Autodesk Fusion 360 part; units mm, degrees
note: some values were not read from the file. Chosen so that the rebuilt part matches the saved one: which pieces of a blend or face edit are solid.
(part 3 of 5)
  circle A747 centre (14.4118, -83.5294) radius 1.5
  circle A748 centre (21.3235, -83.5294) radius 1.5
  circle A749 centre (28.2353, -83.5294) radius 1.5
  circle A750 centre (35.1471, -83.5294) radius 1.5
  circle A751 centre (42.0588, -83.5294) radius 1.5
  circle A752 centre (48.9706, -83.5294) radius 1.5
  circle A753 centre (55.8824, -83.5294) radius 1.5
  circle A754 centre (62.7941, -83.5294) radius 1.5
  circle A755 centre (69.7059, -83.5294) radius 1.5
  circle A756 centre (76.6176, -83.5294) radius 1.5
  circle A757 centre (83.5294, -83.5294) radius 1.5
  circle A758 centre (90.4412, -83.5294) radius 1.5
  circle A759 centre (97.3529, -83.5294) radius 1.5
  circle A760 centre (104.2647, -83.5294) radius 1.5
  circle A761 centre (111.1765, -83.5294) radius 1.5
  circle A762 centre (118.0882, -83.5294) radius 1.5
  circle A763 centre (125, -83.5294) radius 1.5
  circle A764 centre (131.9118, -83.5294) radius 1.5
  circle A765 centre (138.8235, -83.5294) radius 1.5
  circle A766 centre (145.7353, -83.5294) radius 1.5
  circle A767 centre (152.6471, -83.5294) radius 1.5
  circle A768 centre (159.5588, -83.5294) radius 1.5
  circle A769 centre (166.4706, -83.5294) radius 1.5
  circle A770 centre (173.3824, -83.5294) radius 1.5
  circle A771 centre (180.2941, -83.5294) radius 1.5
  circle A772 centre (187.2059, -83.5294) radius 1.5
  circle A773 centre (194.1176, -83.5294) radius 1.5
  circle A774 centre (201.0294, -83.5294) radius 1.5
  circle A775 centre (207.9412, -83.5294) radius 1.5
  circle A776 centre (214.8529, -83.5294) radius 1.5
  circle A777 centre (221.7647, -83.5294) radius 1.5
  circle A778 centre (228.6765, -83.5294) radius 1.5
  circle A779 centre (235.5882, -83.5294) radius 1.5
  circle A780 centre (242.5, -83.5294) radius 1.5
  circle A781 centre (14.4118, -90.4412) radius 1.5
  circle A782 centre (21.3235, -90.4412) radius 1.5
  circle A783 centre (28.2353, -90.4412) radius 1.5
  circle A784 centre (35.1471, -90.4412) radius 1.5
  circle A785 centre (42.0588, -90.4412) radius 1.5
  circle A786 centre (48.9706, -90.4412) radius 1.5
  circle A787 centre (55.8824, -90.4412) radius 1.5
  circle A788 centre (62.7941, -90.4412) radius 1.5
  circle A789 centre (69.7059, -90.4412) radius 1.5
  circle A790 centre (76.6176, -90.4412) radius 1.5
  circle A791 centre (83.5294, -90.4412) radius 1.5
  circle A792 centre (90.4412, -90.4412) radius 1.5
  circle A793 centre (97.3529, -90.4412) radius 1.5
  circle A794 centre (104.2647, -90.4412) radius 1.5
  circle A795 centre (111.1765, -90.4412) radius 1.5
  circle A796 centre (118.0882, -90.4412) radius 1.5
  circle A797 centre (125, -90.4412) radius 1.5
  circle A798 centre (131.9118, -90.4412) radius 1.5
  circle A799 centre (138.8235, -90.4412) radius 1.5
  circle A800 centre (145.7353, -90.4412) radius 1.5
  circle A801 centre (152.6471, -90.4412) radius 1.5
  circle A802 centre (159.5588, -90.4412) radius 1.5
  circle A803 centre (166.4706, -90.4412) radius 1.5
  circle A804 centre (173.3824, -90.4412) radius 1.5
  circle A805 centre (180.2941, -90.4412) radius 1.5
  circle A806 centre (187.2059, -90.4412) radius 1.5
  circle A807 centre (194.1176, -90.4412) radius 1.5
  circle A808 centre (201.0294, -90.4412) radius 1.5
  circle A809 centre (207.9412, -90.4412) radius 1.5
  circle A810 centre (214.8529, -90.4412) radius 1.5
  circle A811 centre (221.7647, -90.4412) radius 1.5
  circle A812 centre (228.6765, -90.4412) radius 1.5
  circle A813 centre (235.5882, -90.4412) radius 1.5
  circle A814 centre (242.5, -90.4412) radius 1.5
  circle A815 centre (14.4118, -97.3529) radius 1.5
  circle A816 centre (21.3235, -97.3529) radius 1.5
  circle A817 centre (28.2353, -97.3529) radius 1.5
  circle A818 centre (35.1471, -97.3529) radius 1.5
  circle A819 centre (42.0588, -97.3529) radius 1.5
  circle A820 centre (48.9706, -97.3529) radius 1.5
  circle A821 centre (55.8824, -97.3529) radius 1.5
  circle A822 centre (62.7941, -97.3529) radius 1.5
  circle A823 centre (69.7059, -97.3529) radius 1.5
  circle A824 centre (76.6176, -97.3529) radius 1.5
  circle A825 centre (83.5294, -97.3529) radius 1.5
  circle A826 centre (90.4412, -97.3529) radius 1.5
  circle A827 centre (97.3529, -97.3529) radius 1.5
  circle A828 centre (104.2647, -97.3529) radius 1.5
  circle A829 centre (111.1765, -97.3529) radius 1.5
  circle A830 centre (118.0882, -97.3529) radius 1.5
  circle A831 centre (125, -97.3529) radius 1.5
  circle A832 centre (131.9118, -97.3529) radius 1.5
  circle A833 centre (138.8235, -97.3529) radius 1.5
  circle A834 centre (145.7353, -97.3529) radius 1.5
  circle A835 centre (152.6471, -97.3529) radius 1.5
  circle A836 centre (159.5588, -97.3529) radius 1.5
  circle A837 centre (166.4706, -97.3529) radius 1.5
  circle A838 centre (173.3824, -97.3529) radius 1.5
  circle A839 centre (180.2941, -97.3529) radius 1.5
  circle A840 centre (187.2059, -97.3529) radius 1.5
  circle A841 centre (194.1176, -97.3529) radius 1.5
  circle A842 centre (201.0294, -97.3529) radius 1.5
  circle A843 centre (207.9412, -97.3529) radius 1.5
  circle A844 centre (214.8529, -97.3529) radius 1.5
  circle A845 centre (221.7647, -97.3529) radius 1.5
  circle A846 centre (228.6765, -97.3529) radius 1.5
  circle A847 centre (235.5882, -97.3529) radius 1.5
  circle A848 centre (242.5, -97.3529) radius 1.5
  circle A849 centre (14.4118, -104.2647) radius 1.5
  circle A850 centre (21.3235, -104.2647) radius 1.5
  circle A851 centre (28.2353, -104.2647) radius 1.5
  circle A852 centre (35.1471, -104.2647) radius 1.5
  circle A853 centre (42.0588, -104.2647) radius 1.5
  circle A854 centre (48.9706, -104.2647) radius 1.5
  circle A855 centre (55.8824, -104.2647) radius 1.5
  circle A856 centre (62.7941, -104.2647) radius 1.5
  circle A857 centre (69.7059, -104.2647) radius 1.5
  circle A858 centre (76.6176, -104.2647) radius 1.5
  circle A859 centre (83.5294, -104.2647) radius 1.5
  circle A860 centre (90.4412, -104.2647) radius 1.5
  circle A861 centre (97.3529, -104.2647) radius 1.5
  circle A862 centre (104.2647, -104.2647) radius 1.5
  circle A863 centre (111.1765, -104.2647) radius 1.5
  circle A864 centre (118.0882, -104.2647) radius 1.5
  circle A865 centre (125, -104.2647) radius 1.5
  circle A866 centre (131.9118, -104.2647) radius 1.5
  circle A867 centre (138.8235, -104.2647) radius 1.5
  circle A868 centre (145.7353, -104.2647) radius 1.5
  circle A869 centre (152.6471, -104.2647) radius 1.5
  circle A870 centre (159.5588, -104.2647) radius 1.5
  circle A871 centre (166.4706, -104.2647) radius 1.5
  circle A872 centre (173.3824, -104.2647) radius 1.5
  circle A873 centre (180.2941, -104.2647) radius 1.5
  circle A874 centre (187.2059, -104.2647) radius 1.5
  circle A875 centre (194.1176, -104.2647) radius 1.5
  circle A876 centre (201.0294, -104.2647) radius 1.5
  circle A877 centre (207.9412, -104.2647) radius 1.5
  circle A878 centre (214.8529, -104.2647) radius 1.5
  circle A879 centre (221.7647, -104.2647) radius 1.5
  circle A880 centre (228.6765, -104.2647) radius 1.5
  circle A881 centre (235.5882, -104.2647) radius 1.5
  circle A882 centre (242.5, -104.2647) radius 1.5
  circle A883 centre (14.4118, -111.1765) radius 1.5
  circle A884 centre (21.3235, -111.1765) radius 1.5
  circle A885 centre (28.2353, -111.1765) radius 1.5
  circle A886 centre (35.1471, -111.1765) radius 1.5
  circle A887 centre (42.0588, -111.1765) radius 1.5
  circle A888 centre (48.9706, -111.1765) radius 1.5
  circle A889 centre (55.8824, -111.1765) radius 1.5
  circle A890 centre (62.7941, -111.1765) radius 1.5
  circle A891 centre (69.7059, -111.1765) radius 1.5
  circle A892 centre (76.6176, -111.1765) radius 1.5
  circle A893 centre (83.5294, -111.1765) radius 1.5
  circle A894 centre (90.4412, -111.1765) radius 1.5
  circle A895 centre (97.3529, -111.1765) radius 1.5
  circle A896 centre (104.2647, -111.1765) radius 1.5
  circle A897 centre (111.1765, -111.1765) radius 1.5
  circle A898 centre (118.0882, -111.1765) radius 1.5
  circle A899 centre (125, -111.1765) radius 1.5
  circle A900 centre (131.9118, -111.1765) radius 1.5
  circle A901 centre (138.8235, -111.1765) radius 1.5
  circle A902 centre (145.7353, -111.1765) radius 1.5
  circle A903 centre (152.6471, -111.1765) radius 1.5
  circle A904 centre (159.5588, -111.1765) radius 1.5
  circle A905 centre (166.4706, -111.1765) radius 1.5
  circle A906 centre (173.3824, -111.1765) radius 1.5
  circle A907 centre (180.2941, -111.1765) radius 1.5
  circle A908 centre (187.2059, -111.1765) radius 1.5
  circle A909 centre (194.1176, -111.1765) radius 1.5
  circle A910 centre (201.0294, -111.1765) radius 1.5
  circle A911 centre (207.9412, -111.1765) radius 1.5
  circle A912 centre (214.8529, -111.1765) radius 1.5
  circle A913 centre (221.7647, -111.1765) radius 1.5
  circle A914 centre (228.6765, -111.1765) radius 1.5
  circle A915 centre (235.5882, -111.1765) radius 1.5
  circle A916 centre (242.5, -111.1765) radius 1.5
  circle A917 centre (14.4118, -118.0882) radius 1.5
  circle A918 centre (21.3235, -118.0882) radius 1.5
  circle A919 centre (28.2353, -118.0882) radius 1.5
  circle A920 centre (35.1471, -118.0882) radius 1.5
  circle A921 centre (42.0588, -118.0882) radius 1.5
  circle A922 centre (48.9706, -118.0882) radius 1.5
  circle A923 centre (55.8824, -118.0882) radius 1.5
  circle A924 centre (62.7941, -118.0882) radius 1.5
  circle A925 centre (69.7059, -118.0882) radius 1.5
  circle A926 centre (76.6176, -118.0882) radius 1.5
  circle A927 centre (83.5294, -118.0882) radius 1.5
  circle A928 centre (90.4412, -118.0882) radius 1.5
  circle A929 centre (97.3529, -118.0882) radius 1.5
  circle A930 centre (104.2647, -118.0882) radius 1.5
  circle A931 centre (111.1765, -118.0882) radius 1.5
  circle A932 centre (118.0882, -118.0882) radius 1.5
  circle A933 centre (125, -118.0882) radius 1.5
  circle A934 centre (131.9118, -118.0882) radius 1.5
  circle A935 centre (138.8235, -118.0882) radius 1.5
  circle A936 centre (145.7353, -118.0882) radius 1.5
  circle A937 centre (152.6471, -118.0882) radius 1.5
  circle A938 centre (159.5588, -118.0882) radius 1.5
  circle A939 centre (166.4706, -118.0882) radius 1.5
  circle A940 centre (173.3824, -118.0882) radius 1.5
  circle A941 centre (180.2941, -118.0882) radius 1.5
  circle A942 centre (187.2059, -118.0882) radius 1.5
  circle A943 centre (194.1176, -118.0882) radius 1.5
  circle A944 centre (201.0294, -118.0882) radius 1.5
  circle A945 centre (207.9412, -118.0882) radius 1.5
  circle A946 centre (214.8529, -118.0882) radius 1.5
  circle A947 centre (221.7647, -118.0882) radius 1.5
  circle A948 centre (228.6765, -118.0882) radius 1.5
  circle A949 centre (235.5882, -118.0882) radius 1.5
  circle A950 centre (242.5, -118.0882) radius 1.5
  circle A951 centre (14.4118, -125) radius 1.5
  circle A952 centre (21.3235, -125) radius 1.5
  circle A953 centre (28.2353, -125) radius 1.5
  circle A954 centre (35.1471, -125) radius 1.5
  circle A955 centre (42.0588, -125) radius 1.5
  circle A956 centre (48.9706, -125) radius 1.5
  circle A957 centre (55.8824, -125) radius 1.5
  circle A958 centre (62.7941, -125) radius 1.5
  circle A959 centre (69.7059, -125) radius 1.5
  circle A960 centre (76.6176, -125) radius 1.5
  circle A961 centre (83.5294, -125) radius 1.5
  circle A962 centre (90.4412, -125) radius 1.5
  circle A963 centre (97.3529, -125) radius 1.5
  circle A964 centre (104.2647, -125) radius 1.5
  circle A965 centre (111.1765, -125) radius 1.5
  circle A966 centre (118.0882, -125) radius 1.5
  circle A967 centre (125, -125) radius 1.5
  circle A968 centre (131.9118, -125) radius 1.5
  circle A969 centre (138.8235, -125) radius 1.5
  circle A970 centre (145.7353, -125) radius 1.5
  circle A971 centre (152.6471, -125) radius 1.5
  circle A972 centre (159.5588, -125) radius 1.5
  circle A973 centre (166.4706, -125) radius 1.5
  circle A974 centre (173.3824, -125) radius 1.5
  circle A975 centre (180.2941, -125) radius 1.5
  circle A976 centre (187.2059, -125) radius 1.5
  circle A977 centre (194.1176, -125) radius 1.5
  circle A978 centre (201.0294, -125) radius 1.5
  circle A979 centre (207.9412, -125) radius 1.5
  circle A980 centre (214.8529, -125) radius 1.5
  circle A981 centre (221.7647, -125) radius 1.5
  circle A982 centre (228.6765, -125) radius 1.5
  circle A983 centre (235.5882, -125) radius 1.5
  circle A984 centre (242.5, -125) radius 1.5
  circle A985 centre (14.4118, -131.9118) radius 1.5
  circle A986 centre (21.3235, -131.9118) radius 1.5
  circle A987 centre (28.2353, -131.9118) radius 1.5
  circle A988 centre (35.1471, -131.9118) radius 1.5
  circle A989 centre (42.0588, -131.9118) radius 1.5
  circle A990 centre (48.9706, -131.9118) radius 1.5
  circle A991 centre (55.8824, -131.9118) radius 1.5
  circle A992 centre (62.7941, -131.9118) radius 1.5
  circle A993 centre (69.7059, -131.9118) radius 1.5
  circle A994 centre (76.6176, -131.9118) radius 1.5
  circle A995 centre (83.5294, -131.9118) radius 1.5
  circle A996 centre (90.4412, -131.9118) radius 1.5
  circle A997 centre (97.3529, -131.9118) radius 1.5
  circle A998 centre (104.2647, -131.9118) radius 1.5
  circle A999 centre (111.1765, -131.9118) radius 1.5
  circle A1000 centre (118.0882, -131.9118) radius 1.5
  circle A1001 centre (125, -131.9118) radius 1.5
  circle A1002 centre (131.9118, -131.9118) radius 1.5
  circle A1003 centre (138.8235, -131.9118) radius 1.5
  circle A1004 centre (145.7353, -131.9118) radius 1.5
  circle A1005 centre (152.6471, -131.9118) radius 1.5
  circle A1006 centre (159.5588, -131.9118) radius 1.5
  circle A1007 centre (166.4706, -131.9118) radius 1.5
  circle A1008 centre (173.3824, -131.9118) radius 1.5
  circle A1009 centre (180.2941, -131.9118) radius 1.5
  circle A1010 centre (187.2059, -131.9118) radius 1.5
  circle A1011 centre (194.1176, -131.9118) radius 1.5
  circle A1012 centre (201.0294, -131.9118) radius 1.5
  circle A1013 centre (207.9412, -131.9118) radius 1.5
  circle A1014 centre (214.8529, -131.9118) radius 1.5
  circle A1015 centre (221.7647, -131.9118) radius 1.5
  circle A1016 centre (228.6765, -131.9118) radius 1.5
  circle A1017 centre (235.5882, -131.9118) radius 1.5
  circle A1018 centre (242.5, -131.9118) radius 1.5
  circle A1019 centre (14.4118, -138.8235) radius 1.5
  circle A1020 centre (21.3235, -138.8235) radius 1.5
  circle A1021 centre (28.2353, -138.8235) radius 1.5
  circle A1022 centre (35.1471, -138.8235) radius 1.5
  circle A1023 centre (42.0588, -138.8235) radius 1.5
  circle A1024 centre (48.9706, -138.8235) radius 1.5
  circle A1025 centre (55.8824, -138.8235) radius 1.5
  circle A1026 centre (62.7941, -138.8235) radius 1.5
  circle A1027 centre (69.7059, -138.8235) radius 1.5
  circle A1028 centre (76.6176, -138.8235) radius 1.5
  circle A1029 centre (83.5294, -138.8235) radius 1.5
  circle A1030 centre (90.4412, -138.8235) radius 1.5
  circle A1031 centre (97.3529, -138.8235) radius 1.5
  circle A1032 centre (104.2647, -138.8235) radius 1.5
  circle A1033 centre (111.1765, -138.8235) radius 1.5
  circle A1034 centre (118.0882, -138.8235) radius 1.5
  circle A1035 centre (125, -138.8235) radius 1.5
  circle A1036 centre (131.9118, -138.8235) radius 1.5
  circle A1037 centre (138.8235, -138.8235) radius 1.5
  circle A1038 centre (145.7353, -138.8235) radius 1.5
  circle A1039 centre (152.6471, -138.8235) radius 1.5
  circle A1040 centre (159.5588, -138.8235) radius 1.5
  circle A1041 centre (166.4706, -138.8235) radius 1.5
  circle A1042 centre (173.3824, -138.8235) radius 1.5
  circle A1043 centre (180.2941, -138.8235) radius 1.5
  circle A1044 centre (187.2059, -138.8235) radius 1.5
  circle A1045 centre (194.1176, -138.8235) radius 1.5
  circle A1046 centre (201.0294, -138.8235) radius 1.5
  circle A1047 centre (207.9412, -138.8235) radius 1.5
  circle A1048 centre (214.8529, -138.8235) radius 1.5
  circle A1049 centre (221.7647, -138.8235) radius 1.5
  circle A1050 centre (228.6765, -138.8235) radius 1.5
  circle A1051 centre (235.5882, -138.8235) radius 1.5
  circle A1052 centre (242.5, -138.8235) radius 1.5
  circle A1053 centre (14.4118, -145.7353) radius 1.5
  circle A1054 centre (21.3235, -145.7353) radius 1.5
  circle A1055 centre (28.2353, -145.7353) radius 1.5
  circle A1056 centre (35.1471, -145.7353) radius 1.5
  circle A1057 centre (42.0588, -145.7353) radius 1.5
  circle A1058 centre (48.9706, -145.7353) radius 1.5
  circle A1059 centre (55.8824, -145.7353) radius 1.5
  circle A1060 centre (62.7941, -145.7353) radius 1.5
  circle A1061 centre (69.7059, -145.7353) radius 1.5
  circle A1062 centre (76.6176, -145.7353) radius 1.5
  circle A1063 centre (83.5294, -145.7353) radius 1.5
  circle A1064 centre (90.4412, -145.7353) radius 1.5
  circle A1065 centre (97.3529, -145.7353) radius 1.5
  circle A1066 centre (104.2647, -145.7353) radius 1.5
  circle A1067 centre (111.1765, -145.7353) radius 1.5
  circle A1068 centre (118.0882, -145.7353) radius 1.5
  circle A1069 centre (125, -145.7353) radius 1.5
  circle A1070 centre (131.9118, -145.7353) radius 1.5
  circle A1071 centre (138.8235, -145.7353) radius 1.5
  circle A1072 centre (145.7353, -145.7353) radius 1.5
  circle A1073 centre (152.6471, -145.7353) radius 1.5
  circle A1074 centre (159.5588, -145.7353) radius 1.5
  circle A1075 centre (166.4706, -145.7353) radius 1.5
  circle A1076 centre (173.3824, -145.7353) radius 1.5
  circle A1077 centre (180.2941, -145.7353) radius 1.5
  circle A1078 centre (187.2059, -145.7353) radius 1.5
  circle A1079 centre (194.1176, -145.7353) radius 1.5
  circle A1080 centre (201.0294, -145.7353) radius 1.5
  circle A1081 centre (207.9412, -145.7353) radius 1.5
  circle A1082 centre (214.8529, -145.7353) radius 1.5
  circle A1083 centre (221.7647, -145.7353) radius 1.5
  circle A1084 centre (228.6765, -145.7353) radius 1.5
  circle A1085 centre (235.5882, -145.7353) radius 1.5
  circle A1086 centre (242.5, -145.7353) radius 1.5
  circle A1087 centre (14.4118, -152.6471) radius 1.5
  circle A1088 centre (21.3235, -152.6471) radius 1.5
  circle A1089 centre (28.2353, -152.6471) radius 1.5
  circle A1090 centre (35.1471, -152.6471) radius 1.5
  circle A1091 centre (42.0588, -152.6471) radius 1.5
  circle A1092 centre (48.9706, -152.6471) radius 1.5
  circle A1093 centre (55.8824, -152.6471) radius 1.5
  circle A1094 centre (62.7941, -152.6471) radius 1.5
  circle A1095 centre (69.7059, -152.6471) radius 1.5
  circle A1096 centre (76.6176, -152.6471) radius 1.5
  circle A1097 centre (83.5294, -152.6471) radius 1.5
  circle A1098 centre (90.4412, -152.6471) radius 1.5
  circle A1099 centre (97.3529, -152.6471) radius 1.5
  circle A1100 centre (104.2647, -152.6471) radius 1.5
  circle A1101 centre (111.1765, -152.6471) radius 1.5
  circle A1102 centre (118.0882, -152.6471) radius 1.5
  circle A1103 centre (125, -152.6471) radius 1.5
  circle A1104 centre (131.9118, -152.6471) radius 1.5
  circle A1105 centre (138.8235, -152.6471) radius 1.5
  circle A1106 centre (145.7353, -152.6471) radius 1.5
  circle A1107 centre (152.6471, -152.6471) radius 1.5
  circle A1108 centre (159.5588, -152.6471) radius 1.5
  circle A1109 centre (166.4706, -152.6471) radius 1.5
  circle A1110 centre (173.3824, -152.6471) radius 1.5
  circle A1111 centre (180.2941, -152.6471) radius 1.5
  circle A1112 centre (187.2059, -152.6471) radius 1.5
  circle A1113 centre (194.1176, -152.6471) radius 1.5
  circle A1114 centre (201.0294, -152.6471) radius 1.5
  circle A1115 centre (207.9412, -152.6471) radius 1.5
  circle A1116 centre (214.8529, -152.6471) radius 1.5
  circle A1117 centre (221.7647, -152.6471) radius 1.5
  circle A1118 centre (228.6765, -152.6471) radius 1.5
  circle A1119 centre (235.5882, -152.6471) radius 1.5
  circle A1120 centre (242.5, -152.6471) radius 1.5
  circle A1121 centre (14.4118, -159.5588) radius 1.5
  circle A1122 centre (21.3235, -159.5588) radius 1.5
  circle A1123 centre (28.2353, -159.5588) radius 1.5
  circle A1124 centre (35.1471, -159.5588) radius 1.5
  circle A1125 centre (42.0588, -159.5588) radius 1.5
  circle A1126 centre (48.9706, -159.5588) radius 1.5
  circle A1127 centre (55.8824, -159.5588) radius 1.5
  circle A1128 centre (62.7941, -159.5588) radius 1.5
  circle A1129 centre (69.7059, -159.5588) radius 1.5
  circle A1130 centre (76.6176, -159.5588) radius 1.5
  circle A1131 centre (83.5294, -159.5588) radius 1.5
  circle A1132 centre (90.4412, -159.5588) radius 1.5
  circle A1133 centre (97.3529, -159.5588) radius 1.5
  circle A1134 centre (104.2647, -159.5588) radius 1.5
  circle A1135 centre (111.1765, -159.5588) radius 1.5
  circle A1136 centre (118.0882, -159.5588) radius 1.5
  circle A1137 centre (125, -159.5588) radius 1.5
  circle A1138 centre (131.9118, -159.5588) radius 1.5
  circle A1139 centre (138.8235, -159.5588) radius 1.5
  circle A1140 centre (145.7353, -159.5588) radius 1.5
  circle A1141 centre (152.6471, -159.5588) radius 1.5
  circle A1142 centre (159.5588, -159.5588) radius 1.5
  circle A1143 centre (166.4706, -159.5588) radius 1.5
  circle A1144 centre (173.3824, -159.5588) radius 1.5
  circle A1145 centre (180.2941, -159.5588) radius 1.5
  circle A1146 centre (187.2059, -159.5588) radius 1.5
  circle A1147 centre (194.1176, -159.5588) radius 1.5
  circle A1148 centre (201.0294, -159.5588) radius 1.5
  circle A1149 centre (207.9412, -159.5588) radius 1.5
  circle A1150 centre (214.8529, -159.5588) radius 1.5
  circle A1151 centre (221.7647, -159.5588) radius 1.5
  circle A1152 centre (228.6765, -159.5588) radius 1.5
  circle A1153 centre (235.5882, -159.5588) radius 1.5
  circle A1154 centre (242.5, -159.5588) radius 1.5
  circle A1155 centre (14.4118, -166.4706) radius 1.5
  circle A1156 centre (21.3235, -166.4706) radius 1.5
  circle A1157 centre (28.2353, -166.4706) radius 1.5
  circle A1158 centre (35.1471, -166.4706) radius 1.5
  circle A1159 centre (42.0588, -166.4706) radius 1.5
  circle A1160 centre (48.9706, -166.4706) radius 1.5
  circle A1161 centre (55.8824, -166.4706) radius 1.5
  circle A1162 centre (62.7941, -166.4706) radius 1.5
  circle A1163 centre (69.7059, -166.4706) radius 1.5
  circle A1164 centre (76.6176, -166.4706) radius 1.5
  circle A1165 centre (83.5294, -166.4706) radius 1.5
  circle A1166 centre (90.4412, -166.4706) radius 1.5
  circle A1167 centre (97.3529, -166.4706) radius 1.5
  circle A1168 centre (104.2647, -166.4706) radius 1.5
  circle A1169 centre (111.1765, -166.4706) radius 1.5
  circle A1170 centre (118.0882, -166.4706) radius 1.5
  circle A1171 centre (125, -166.4706) radius 1.5
  circle A1172 centre (131.9118, -166.4706) radius 1.5
  circle A1173 centre (138.8235, -166.4706) radius 1.5
  circle A1174 centre (145.7353, -166.4706) radius 1.5
  circle A1175 centre (152.6471, -166.4706) radius 1.5
  circle A1176 centre (159.5588, -166.4706) radius 1.5
  circle A1177 centre (166.4706, -166.4706) radius 1.5
  circle A1178 centre (173.3824, -166.4706) radius 1.5
  circle A1179 centre (180.2941, -166.4706) radius 1.5
  circle A1180 centre (187.2059, -166.4706) radius 1.5
  circle A1181 centre (194.1176, -166.4706) radius 1.5
  circle A1182 centre (201.0294, -166.4706) radius 1.5
  circle A1183 centre (207.9412, -166.4706) radius 1.5
  circle A1184 centre (214.8529, -166.4706) radius 1.5
  circle A1185 centre (221.7647, -166.4706) radius 1.5
  circle A1186 centre (228.6765, -166.4706) radius 1.5
  circle A1187 centre (235.5882, -166.4706) radius 1.5
  circle A1188 centre (242.5, -166.4706) radius 1.5
  circle A1189 centre (14.4118, -173.3824) radius 1.5
  circle A1190 centre (21.3235, -173.3824) radius 1.5
  circle A1191 centre (28.2353, -173.3824) radius 1.5
  circle A1192 centre (35.1471, -173.3824) radius 1.5
  circle A1193 centre (42.0588, -173.3824) radius 1.5
  circle A1194 centre (48.9706, -173.3824) radius 1.5
  circle A1195 centre (55.8824, -173.3824) radius 1.5
  circle A1196 centre (62.7941, -173.3824) radius 1.5
  circle A1197 centre (69.7059, -173.3824) radius 1.5
  circle A1198 centre (76.6176, -173.3824) radius 1.5
  circle A1199 centre (83.5294, -173.3824) radius 1.5
  circle A1200 centre (90.4412, -173.3824) radius 1.5
  circle A1201 centre (97.3529, -173.3824) radius 1.5
  circle A1202 centre (104.2647, -173.3824) radius 1.5
  circle A1203 centre (111.1765, -173.3824) radius 1.5
  circle A1204 centre (118.0882, -173.3824) radius 1.5
  circle A1205 centre (125, -173.3824) radius 1.5
  circle A1206 centre (131.9118, -173.3824) radius 1.5
  circle A1207 centre (138.8235, -173.3824) radius 1.5
  circle A1208 centre (145.7353, -173.3824) radius 1.5
  circle A1209 centre (152.6471, -173.3824) radius 1.5
  circle A1210 centre (159.5588, -173.3824) radius 1.5
  circle A1211 centre (166.4706, -173.3824) radius 1.5
  circle A1212 centre (173.3824, -173.3824) radius 1.5
  circle A1213 centre (180.2941, -173.3824) radius 1.5
  circle A1214 centre (187.2059, -173.3824) radius 1.5
  circle A1215 centre (194.1176, -173.3824) radius 1.5
  circle A1216 centre (201.0294, -173.3824) radius 1.5
  circle A1217 centre (207.9412, -173.3824) radius 1.5
  circle A1218 centre (214.8529, -173.3824) radius 1.5
  circle A1219 centre (221.7647, -173.3824) radius 1.5
  circle A1220 centre (228.6765, -173.3824) radius 1.5
  circle A1221 centre (235.5882, -173.3824) radius 1.5
  circle A1222 centre (242.5, -173.3824) radius 1.5
  circle A1223 centre (14.4118, -180.2941) radius 1.5
  circle A1224 centre (21.3235, -180.2941) radius 1.5
  circle A1225 centre (28.2353, -180.2941) radius 1.5
  circle A1226 centre (35.1471, -180.2941) radius 1.5
  circle A1227 centre (42.0588, -180.2941) radius 1.5
  circle A1228 centre (48.9706, -180.2941) radius 1.5
  circle A1229 centre (55.8824, -180.2941) radius 1.5
  circle A1230 centre (62.7941, -180.2941) radius 1.5
  circle A1231 centre (69.7059, -180.2941) radius 1.5
  circle A1232 centre (76.6176, -180.2941) radius 1.5
  circle A1233 centre (83.5294, -180.2941) radius 1.5
  circle A1234 centre (90.4412, -180.2941) radius 1.5
  circle A1235 centre (97.3529, -180.2941) radius 1.5
  circle A1236 centre (104.2647, -180.2941) radius 1.5
  circle A1237 centre (111.1765, -180.2941) radius 1.5
  circle A1238 centre (118.0882, -180.2941) radius 1.5
  circle A1239 centre (125, -180.2941) radius 1.5
  circle A1240 centre (131.9118, -180.2941) radius 1.5
  circle A1241 centre (138.8235, -180.2941) radius 1.5
  circle A1242 centre (145.7353, -180.2941) radius 1.5
  circle A1243 centre (152.6471, -180.2941) radius 1.5
  circle A1244 centre (159.5588, -180.2941) radius 1.5
  circle A1245 centre (166.4706, -180.2941) radius 1.5
  circle A1246 centre (173.3824, -180.2941) radius 1.5
  circle A1247 centre (180.2941, -180.2941) radius 1.5
  circle A1248 centre (187.2059, -180.2941) radius 1.5
  circle A1249 centre (194.1176, -180.2941) radius 1.5
  circle A1250 centre (201.0294, -180.2941) radius 1.5
  circle A1251 centre (207.9412, -180.2941) radius 1.5
  circle A1252 centre (214.8529, -180.2941) radius 1.5
  circle A1253 centre (221.7647, -180.2941) radius 1.5
  circle A1254 centre (228.6765, -180.2941) radius 1.5
  circle A1255 centre (235.5882, -180.2941) radius 1.5
  circle A1256 centre (242.5, -180.2941) radius 1.5
  circle A1257 centre (14.4118, -187.2059) radius 1.5
  circle A1258 centre (21.3235, -187.2059) radius 1.5
  circle A1259 centre (28.2353, -187.2059) radius 1.5
  circle A1260 centre (35.1471, -187.2059) radius 1.5
  circle A1261 centre (42.0588, -187.2059) radius 1.5
  circle A1262 centre (48.9706, -187.2059) radius 1.5
  circle A1263 centre (55.8824, -187.2059) radius 1.5
  circle A1264 centre (62.7941, -187.2059) radius 1.5
  circle A1265 centre (69.7059, -187.2059) radius 1.5
  circle A1266 centre (76.6176, -187.2059) radius 1.5
  circle A1267 centre (83.5294, -187.2059) radius 1.5
  circle A1268 centre (90.4412, -187.2059) radius 1.5
  circle A1269 centre (97.3529, -187.2059) radius 1.5
  circle A1270 centre (104.2647, -187.2059) radius 1.5
  circle A1271 centre (111.1765, -187.2059) radius 1.5
  circle A1272 centre (118.0882, -187.2059) radius 1.5
  circle A1273 centre (125, -187.2059) radius 1.5
  circle A1274 centre (131.9118, -187.2059) radius 1.5
  circle A1275 centre (138.8235, -187.2059) radius 1.5
  circle A1276 centre (145.7353, -187.2059) radius 1.5
  circle A1277 centre (152.6471, -187.2059) radius 1.5
  circle A1278 centre (159.5588, -187.2059) radius 1.5
  circle A1279 centre (166.4706, -187.2059) radius 1.5
  circle A1280 centre (173.3824, -187.2059) radius 1.5
  circle A1281 centre (180.2941, -187.2059) radius 1.5
  circle A1282 centre (187.2059, -187.2059) radius 1.5
  circle A1283 centre (194.1176, -187.2059) radius 1.5
  circle A1284 centre (201.0294, -187.2059) radius 1.5
  circle A1285 centre (207.9412, -187.2059) radius 1.5
  circle A1286 centre (214.8529, -187.2059) radius 1.5
  circle A1287 centre (221.7647, -187.2059) radius 1.5
  circle A1288 centre (228.6765, -187.2059) radius 1.5
  circle A1289 centre (235.5882, -187.2059) radius 1.5
  circle A1290 centre (242.5, -187.2059) radius 1.5
  circle A1291 centre (14.4118, -194.1176) radius 1.5
  circle A1292 centre (21.3235, -194.1176) radius 1.5
  circle A1293 centre (28.2353, -194.1176) radius 1.5
  circle A1294 centre (35.1471, -194.1176) radius 1.5
  circle A1295 centre (42.0588, -194.1176) radius 1.5
  circle A1296 centre (48.9706, -194.1176) radius 1.5
  circle A1297 centre (55.8824, -194.1176) radius 1.5
  circle A1298 centre (62.7941, -194.1176) radius 1.5
  circle A1299 centre (69.7059, -194.1176) radius 1.5
  circle A1300 centre (76.6176, -194.1176) radius 1.5
  circle A1301 centre (83.5294, -194.1176) radius 1.5
  circle A1302 centre (90.4412, -194.1176) radius 1.5
  circle A1303 centre (97.3529, -194.1176) radius 1.5
  circle A1304 centre (104.2647, -194.1176) radius 1.5
  circle A1305 centre (111.1765, -194.1176) radius 1.5
  circle A1306 centre (118.0882, -194.1176) radius 1.5
  circle A1307 centre (125, -194.1176) radius 1.5
  circle A1308 centre (131.9118, -194.1176) radius 1.5
  circle A1309 centre (138.8235, -194.1176) radius 1.5
  circle A1310 centre (145.7353, -194.1176) radius 1.5
  circle A1311 centre (152.6471, -194.1176) radius 1.5
  circle A1312 centre (159.5588, -194.1176) radius 1.5
  circle A1313 centre (166.4706, -194.1176) radius 1.5
  circle A1314 centre (173.3824, -194.1176) radius 1.5
  circle A1315 centre (180.2941, -194.1176) radius 1.5
  circle A1316 centre (187.2059, -194.1176) radius 1.5
  circle A1317 centre (194.1176, -194.1176) radius 1.5
  circle A1318 centre (201.0294, -194.1176) radius 1.5
  circle A1319 centre (207.9412, -194.1176) radius 1.5
  circle A1320 centre (214.8529, -194.1176) radius 1.5
  circle A1321 centre (221.7647, -194.1176) radius 1.5
  circle A1322 centre (228.6765, -194.1176) radius 1.5
  circle A1323 centre (235.5882, -194.1176) radius 1.5
  circle A1324 centre (242.5, -194.1176) radius 1.5
  circle A1325 centre (14.4118, -201.0294) radius 1.5
  circle A1326 centre (21.3235, -201.0294) radius 1.5
  circle A1327 centre (28.2353, -201.0294) radius 1.5
  circle A1328 centre (35.1471, -201.0294) radius 1.5
  circle A1329 centre (42.0588, -201.0294) radius 1.5
  circle A1330 centre (48.9706, -201.0294) radius 1.5
  circle A1331 centre (55.8824, -201.0294) radius 1.5
  circle A1332 centre (62.7941, -201.0294) radius 1.5
  circle A1333 centre (69.7059, -201.0294) radius 1.5
  circle A1334 centre (76.6176, -201.0294) radius 1.5
  circle A1335 centre (83.5294, -201.0294) radius 1.5
  circle A1336 centre (90.4412, -201.0294) radius 1.5
  circle A1337 centre (97.3529, -201.0294) radius 1.5
  circle A1338 centre (104.2647, -201.0294) radius 1.5
  circle A1339 centre (111.1765, -201.0294) radius 1.5
  circle A1340 centre (118.0882, -201.0294) radius 1.5
  circle A1341 centre (125, -201.0294) radius 1.5
  circle A1342 centre (131.9118, -201.0294) radius 1.5
  circle A1343 centre (138.8235, -201.0294) radius 1.5
  circle A1344 centre (145.7353, -201.0294) radius 1.5
  circle A1345 centre (152.6471, -201.0294) radius 1.5
  circle A1346 centre (159.5588, -201.0294) radius 1.5
  circle A1347 centre (166.4706, -201.0294) radius 1.5
  circle A1348 centre (173.3824, -201.0294) radius 1.5
  circle A1349 centre (180.2941, -201.0294) radius 1.5
  circle A1350 centre (187.2059, -201.0294) radius 1.5
  circle A1351 centre (194.1176, -201.0294) radius 1.5
  circle A1352 centre (201.0294, -201.0294) radius 1.5
  circle A1353 centre (207.9412, -201.0294) radius 1.5
  circle A1354 centre (214.8529, -201.0294) radius 1.5
  circle A1355 centre (221.7647, -201.0294) radius 1.5
  circle A1356 centre (228.6765, -201.0294) radius 1.5
  circle A1357 centre (235.5882, -201.0294) radius 1.5
  circle A1358 centre (242.5, -201.0294) radius 1.5
  circle A1359 centre (14.4118, -207.9412) radius 1.5
  circle A1360 centre (21.3235, -207.9412) radius 1.5
  circle A1361 centre (28.2353, -207.9412) radius 1.5
  circle A1362 centre (35.1471, -207.9412) radius 1.5
  circle A1363 centre (42.0588, -207.9412) radius 1.5
  circle A1364 centre (48.9706, -207.9412) radius 1.5
  circle A1365 centre (55.8824, -207.9412) radius 1.5
  circle A1366 centre (62.7941, -207.9412) radius 1.5
  circle A1367 centre (69.7059, -207.9412) radius 1.5
  circle A1368 centre (76.6176, -207.9412) radius 1.5
  circle A1369 centre (83.5294, -207.9412) radius 1.5
  circle A1370 centre (90.4412, -207.9412) radius 1.5
  circle A1371 centre (97.3529, -207.9412) radius 1.5
  circle A1372 centre (104.2647, -207.9412) radius 1.5
  circle A1373 centre (111.1765, -207.9412) radius 1.5
  circle A1374 centre (118.0882, -207.9412) radius 1.5
  circle A1375 centre (125, -207.9412) radius 1.5
  circle A1376 centre (131.9118, -207.9412) radius 1.5
  circle A1377 centre (138.8235, -207.9412) radius 1.5
  circle A1378 centre (145.7353, -207.9412) radius 1.5
  circle A1379 centre (152.6471, -207.9412) radius 1.5
  circle A1380 centre (159.5588, -207.9412) radius 1.5
  circle A1381 centre (166.4706, -207.9412) radius 1.5
  circle A1382 centre (173.3824, -207.9412) radius 1.5
  circle A1383 centre (180.2941, -207.9412) radius 1.5
  circle A1384 centre (187.2059, -207.9412) radius 1.5
  circle A1385 centre (194.1176, -207.9412) radius 1.5
  circle A1386 centre (201.0294, -207.9412) radius 1.5
  circle A1387 centre (207.9412, -207.9412) radius 1.5
  circle A1388 centre (214.8529, -207.9412) radius 1.5
  circle A1389 centre (221.7647, -207.9412) radius 1.5
  circle A1390 centre (228.6765, -207.9412) radius 1.5
  circle A1391 centre (235.5882, -207.9412) radius 1.5
  circle A1392 centre (242.5, -207.9412) radius 1.5
  circle A1393 centre (14.4118, -214.8529) radius 1.5
  circle A1394 centre (21.3235, -214.8529) radius 1.5
  circle A1395 centre (28.2353, -214.8529) radius 1.5
  circle A1396 centre (35.1471, -214.8529) radius 1.5
  circle A1397 centre (42.0588, -214.8529) radius 1.5
  circle A1398 centre (48.9706, -214.8529) radius 1.5
  circle A1399 centre (55.8824, -214.8529) radius 1.5
  circle A1400 centre (62.7941, -214.8529) radius 1.5
  circle A1401 centre (69.7059, -214.8529) radius 1.5
  circle A1402 centre (76.6176, -214.8529) radius 1.5
  circle A1403 centre (83.5294, -214.8529) radius 1.5
  circle A1404 centre (90.4412, -214.8529) radius 1.5
  circle A1405 centre (97.3529, -214.8529) radius 1.5
  circle A1406 centre (104.2647, -214.8529) radius 1.5
  circle A1407 centre (111.1765, -214.8529) radius 1.5
  circle A1408 centre (118.0882, -214.8529) radius 1.5
  circle A1409 centre (125, -214.8529) radius 1.5
  circle A1410 centre (131.9118, -214.8529) radius 1.5
  circle A1411 centre (138.8235, -214.8529) radius 1.5
  circle A1412 centre (145.7353, -214.8529) radius 1.5
  circle A1413 centre (152.6471, -214.8529) radius 1.5
  circle A1414 centre (159.5588, -214.8529) radius 1.5
  circle A1415 centre (166.4706, -214.8529) radius 1.5
  circle A1416 centre (173.3824, -214.8529) radius 1.5
  circle A1417 centre (180.2941, -214.8529) radius 1.5
  circle A1418 centre (187.2059, -214.8529) radius 1.5
  circle A1419 centre (194.1176, -214.8529) radius 1.5
  circle A1420 centre (201.0294, -214.8529) radius 1.5
  circle A1421 centre (207.9412, -214.8529) radius 1.5
  circle A1422 centre (214.8529, -214.8529) radius 1.5
  circle A1423 centre (221.7647, -214.8529) radius 1.5
  circle A1424 centre (235.5882, -214.8529) radius 1.5
  circle A1425 centre (242.5, -214.8529) radius 1.5
  circle A1426 centre (14.4118, -221.7647) radius 1.5
  circle A1427 centre (21.3235, -221.7647) radius 1.5
  circle A1428 centre (28.2353, -221.7647) radius 1.5
  circle A1429 centre (35.1471, -221.7647) radius 1.5
  circle A1430 centre (42.0588, -221.7647) radius 1.5
  circle A1431 centre (48.9706, -221.7647) radius 1.5
  circle A1432 centre (55.8824, -221.7647) radius 1.5
  circle A1433 centre (62.7941, -221.7647) radius 1.5
  circle A1434 centre (69.7059, -221.7647) radius 1.5
  circle A1435 centre (76.6176, -221.7647) radius 1.5
  circle A1436 centre (83.5294, -221.7647) radius 1.5
  circle A1437 centre (90.4412, -221.7647) radius 1.5
  circle A1438 centre (97.3529, -221.7647) radius 1.5
  circle A1439 centre (104.2647, -221.7647) radius 1.5
  circle A1440 centre (111.1765, -221.7647) radius 1.5
  circle A1441 centre (118.0882, -221.7647) radius 1.5
  circle A1442 centre (125, -221.7647) radius 1.5
  circle A1443 centre (131.9118, -221.7647) radius 1.5
  circle A1444 centre (138.8235, -221.7647) radius 1.5
  circle A1445 centre (145.7353, -221.7647) radius 1.5
  circle A1446 centre (152.6471, -221.7647) radius 1.5
  circle A1447 centre (159.5588, -221.7647) radius 1.5
  circle A1448 centre (166.4706, -221.7647) radius 1.5
  circle A1449 centre (173.3824, -221.7647) radius 1.5
  circle A1450 centre (180.2941, -221.7647) radius 1.5
  circle A1451 centre (187.2059, -221.7647) radius 1.5
  circle A1452 centre (194.1176, -221.7647) radius 1.5
  circle A1453 centre (201.0294, -221.7647) radius 1.5
  circle A1454 centre (207.9412, -221.7647) radius 1.5
  circle A1455 centre (214.8529, -221.7647) radius 1.5
  circle A1456 centre (221.7647, -221.7647) radius 1.5
  circle A1457 centre (235.5882, -221.7647) radius 1.5
  circle A1458 centre (242.5, -221.7647) radius 1.5
  circle A1459 centre (14.4118, -228.6765) radius 1.5
  circle A1460 centre (21.3235, -228.6765) radius 1.5
  circle A1461 centre (28.2353, -228.6765) radius 1.5
  circle A1462 centre (35.1471, -228.6765) radius 1.5
  circle A1463 centre (42.0588, -228.6765) radius 1.5
  circle A1464 centre (48.9706, -228.6765) radius 1.5
  circle A1465 centre (55.8824, -228.6765) radius 1.5
  circle A1466 centre (62.7941, -228.6765) radius 1.5
  circle A1467 centre (69.7059, -228.6765) radius 1.5
  circle A1468 centre (76.6176, -228.6765) radius 1.5
  circle A1469 centre (83.5294, -228.6765) radius 1.5
  circle A1470 centre (90.4412, -228.6765) radius 1.5
  circle A1471 centre (97.3529, -228.6765) radius 1.5
  circle A1472 centre (104.2647, -228.6765) radius 1.5
  circle A1473 centre (111.1765, -228.6765) radius 1.5
  circle A1474 centre (118.0882, -228.6765) radius 1.5
  circle A1475 centre (125, -228.6765) radius 1.5
  circle A1476 centre (131.9118, -228.6765) radius 1.5
  circle A1477 centre (138.8235, -228.6765) radius 1.5
  circle A1478 centre (145.7353, -228.6765) radius 1.5
  circle A1479 centre (152.6471, -228.6765) radius 1.5
  circle A1480 centre (159.5588, -228.6765) radius 1.5
  circle A1481 centre (166.4706, -228.6765) radius 1.5
  circle A1482 centre (173.3824, -228.6765) radius 1.5
  circle A1483 centre (180.2941, -228.6765) radius 1.5
  circle A1484 centre (187.2059, -228.6765) radius 1.5
  circle A1485 centre (194.1176, -228.6765) radius 1.5
  circle A1486 centre (201.0294, -228.6765) radius 1.5
  circle A1487 centre (207.9412, -228.6765) radius 1.5
  circle A1488 centre (214.8529, -228.6765) radius 1.5
  circle A1489 centre (221.7647, -228.6765) radius 1.5
  circle A1490 centre (235.5882, -228.6765) radius 1.5
  circle A1491 centre (242.5, -228.6765) radius 1.5
  circle A1492 centre (14.4118, -235.5882) radius 1.5
  circle A1493 centre (21.3235, -235.5882) radius 1.5
  circle A1494 centre (28.2353, -235.5882) radius 1.5
  circle A1495 centre (35.1471, -235.5882) radius 1.5
  circle A1496 centre (42.0588, -235.5882) radius 1.5
  circle A1497 centre (48.9706, -235.5882) radius 1.5
  circle A1498 centre (55.8824, -235.5882) radius 1.5
  circle A1499 centre (62.7941, -235.5882) radius 1.5
  circle A1500 centre (69.7059, -235.5882) radius 1.5
  circle A1501 centre (76.6176, -235.5882) radius 1.5
  circle A1502 centre (83.5294, -235.5882) radius 1.5
  circle A1503 centre (90.4412, -235.5882) radius 1.5
  circle A1504 centre (97.3529, -235.5882) radius 1.5
  circle A1505 centre (104.2647, -235.5882) radius 1.5
  circle A1506 centre (111.1765, -235.5882) radius 1.5
  circle A1507 centre (118.0882, -235.5882) radius 1.5
  circle A1508 centre (125, -235.5882) radius 1.5
  circle A1509 centre (131.9118, -235.5882) radius 1.5
  circle A1510 centre (138.8235, -235.5882) radius 1.5
  circle A1511 centre (145.7353, -235.5882) radius 1.5
  circle A1512 centre (152.6471, -235.5882) radius 1.5
  circle A1513 centre (159.5588, -235.5882) radius 1.5
  circle A1514 centre (166.4706, -235.5882) radius 1.5
  circle A1515 centre (173.3824, -235.5882) radius 1.5
  circle A1516 centre (180.2941, -235.5882) radius 1.5
  circle A1517 centre (187.2059, -235.5882) radius 1.5
  circle A1518 centre (194.1176, -235.5882) radius 1.5
  circle A1519 centre (201.0294, -235.5882) radius 1.5
  circle A1520 centre (207.9412, -235.5882) radius 1.5
  circle A1521 centre (214.8529, -235.5882) radius 1.5
  circle A1522 centre (221.7647, -235.5882) radius 1.5
  circle A1523 centre (235.5882, -235.5882) radius 1.5
  circle A1524 centre (242.5, -235.5882) radius 1.5
  circle A1525 centre (14.4118, -242.5) radius 1.5
  circle A1526 centre (21.3235, -242.5) radius 1.5
  circle A1527 centre (28.2353, -242.5) radius 1.5
  circle A1528 centre (35.1471, -242.5) radius 1.5
  circle A1529 centre (42.0588, -242.5) radius 1.5
  circle A1530 centre (48.9706, -242.5) radius 1.5
  circle A1531 centre (55.8824, -242.5) radius 1.5
  circle A1532 centre (62.7941, -242.5) radius 1.5
  circle A1533 centre (69.7059, -242.5) radius 1.5
  circle A1534 centre (76.6176, -242.5) radius 1.5
  circle A1535 centre (83.5294, -242.5) radius 1.5
  circle A1536 centre (90.4412, -242.5) radius 1.5
  circle A1537 centre (97.3529, -242.5) radius 1.5
  circle A1538 centre (104.2647, -242.5) radius 1.5
  circle A1539 centre (111.1765, -242.5) radius 1.5
  circle A1540 centre (118.0882, -242.5) radius 1.5
  circle A1541 centre (125, -242.5) radius 1.5
  circle A1542 centre (131.9118, -242.5) radius 1.5
  circle A1543 centre (138.8235, -242.5) radius 1.5
  circle A1544 centre (145.7353, -242.5) radius 1.5
  circle A1545 centre (152.6471, -242.5) radius 1.5
  circle A1546 centre (159.5588, -242.5) radius 1.5
  circle A1547 centre (166.4706, -242.5) radius 1.5
  circle A1548 centre (173.3824, -242.5) radius 1.5
  circle A1549 centre (180.2941, -242.5) radius 1.5
  circle A1550 centre (187.2059, -242.5) radius 1.5
  circle A1551 centre (194.1176, -242.5) radius 1.5
  circle A1552 centre (201.0294, -242.5) radius 1.5
  circle A1553 centre (207.9412, -242.5) radius 1.5
  circle A1554 centre (214.8529, -242.5) radius 1.5
  circle A1555 centre (221.7647, -242.5) radius 1.5
  circle A1556 centre (235.5882, -242.5) radius 1.5
  circle A1557 centre (242.5, -242.5) radius 1.5
  line L210 (0.2007, 77.9951) -> (0.1004, 42.9426)
  line L211 (-7.8996, 42.9426) -> (0.1004, 42.9426)
  line L212 (250.1004, 352.1103) -> (258.1004, 352.1103)
  line L213 (250.1004, 324.3325) -> (258.1004, 324.3325)
  line L214 (250.1004, 296.5548) -> (258.1004, 296.5548)
  line L215 (250.1004, 268.777) -> (258.1004, 268.777)
  line L216 (250.1004, 240.9992) -> (258.1004, 240.9992)
  line L217 (250.1004, 213.2214) -> (258.1004, 213.2214)
  line L218 (250.1004, 185.4437) -> (258.1004, 185.4437)
  line L219 (250.1004, 157.6659) -> (258.1004, 157.6659)
  line L220 (258.1004, 352.1103) -> (258.1004, 324.3325)
  line L221 (258.1004, 185.4437) -> (258.1004, 157.6659)
  line L222 (258.1004, 296.5548) -> (258.1004, 268.777)
  line L223 (258.1004, 240.9992) -> (258.1004, 213.2214)
  line L224 (250.1004, 296.5548) -> (250.1004, 324.3325)
  line L225 (250.1004, 352.1103) -> (250.1004, 379.8881)
  line L226 (250.1004, 129.8881) -> (250.1004, 157.6659)
  line L227 (250.1004, 185.4437) -> (250.1004, 213.2214)
  line L228 (250.1004, 240.9992) -> (250.1004, 268.777)
  point P0 (7.5, -7.5)
  point P1 (250, -328)
  point P2 (7.5, -265.5)
  point P3 (19.25, -265.5)
  point P4 (19.25, -265.5)
  point P5 (7.5, -274.6667)
  point P6 (7.5, -274.6667)
  point P7 (19.25, -274.6667)
  point P8 (19.25, -274.6667)
  point P9 (-8, 0)
  point P10 (239.5, -268.5)
  point P11 (31, -265.5)
  point P12 (31, -265.5)
  point P13 (42.75, -265.5)
  point P14 (42.75, -265.5)
  point P15 (54.5, -265.5)
  point P16 (54.5, -265.5)
  point P17 (66.25, -265.5)
  point P18 (66.25, -265.5)
  point P19 (78, -265.5)
  point P20 (78, -265.5)
  point P21 (89.75, -265.5)
  point P22 (89.75, -265.5)
  point P23 (101.5, -265.5)
  point P24 (101.5, -265.5)
  point P25 (125, -265.5)
  point P26 (125, -265.5)
  point P27 (136.75, -265.5)
  point P28 (136.75, -265.5)
  point P29 (148.5, -265.5)
  point P30 (148.5, -265.5)
  point P31 (183.75, -265.5)
  point P32 (183.75, -265.5)
  point P33 (195.5, -265.5)
  point P34 (195.5, -265.5)
  point P35 (207.25, -265.5)
  point P36 (207.25, -265.5)
  point P37 (31, -274.6667)
  point P38 (31, -274.6667)
  point P39 (42.75, -274.6667)
  point P40 (42.75, -274.6667)
  point P41 (183.75, -274.6667)
  point P42 (183.75, -274.6667)
  point P43 (195.5, -274.6667)
  point P44 (195.5, -274.6667)
  point P45 (207.25, -274.6667)
  point P46 (207.25, -274.6667)
  point P47 (7.5, -283.8333)
  point P48 (7.5, -283.8333)
  point P49 (19.25, -283.8333)
  point P50 (19.25, -283.8333)
  point P51 (31, -283.8333)
  point P52 (31, -283.8333)
  point P53 (195.5, -283.8333)
  point P54 (195.5, -283.8333)
  point P55 (207.25, -283.8333)
  point P56 (207.25, -283.8333)
  point P57 (7.5, -293)
  point P58 (7.5, -293)
  point P59 (19.25, -293)
  point P60 (19.25, -293)
  point P61 (31, -293)
  point P62 (31, -293)
  point P63 (195.5, -293)
  point P64 (195.5, -293)
  point P65 (207.25, -293)
  point P66 (207.25, -293)
  point P67 (7.5, -302.1667)
  point P68 (7.5, -302.1667)
  point P69 (19.25, -302.1667)
  point P70 (19.25, -302.1667)
  point P71 (31, -302.1667)
  point P72 (31, -302.1667)
  point P73 (42.75, -302.1667)
  point P74 (42.75, -302.1667)
  point P75 (183.75, -302.1667)
  point P76 (183.75, -302.1667)
  point P77 (195.5, -302.1667)
  point P78 (195.5, -302.1667)
  point P79 (207.25, -302.1667)
  point P80 (207.25, -302.1667)
  point P81 (7.5, -311.3333)
  point P82 (7.5, -311.3333)
  point P83 (19.25, -311.3333)
  point P84 (19.25, -311.3333)
  point P85 (31, -311.3333)
  point P86 (31, -311.3333)
  point P87 (42.75, -311.3333)
  point P88 (42.75, -311.3333)
  point P89 (54.5, -311.3333)
  point P90 (54.5, -311.3333)
  point P91 (66.25, -311.3333)
  point P92 (66.25, -311.3333)
  point P93 (78, -311.3333)
  point P94 (78, -311.3333)
  point P95 (89.75, -311.3333)
  point P96 (89.75, -311.3333)
  point P97 (101.5, -311.3333)
  point P98 (101.5, -311.3333)
  point P99 (113.25, -311.3333)
  point P100 (113.25, -311.3333)
  point P101 (125, -311.3333)
  point P102 (125, -311.3333)
  point P103 (136.75, -311.3333)
  point P104 (136.75, -311.3333)
  point P105 (148.5, -311.3333)
  point P106 (148.5, -311.3333)
  point P107 (160.25, -311.3333)
  point P108 (160.25, -311.3333)
  point P109 (172, -311.3333)
  point P110 (172, -311.3333)
  point P111 (183.75, -311.3333)
  point P112 (183.75, -311.3333)
  point P113 (195.5, -311.3333)
  point P114 (195.5, -311.3333)
  point P115 (207.25, -311.3333)
  point P116 (207.25, -311.3333)
  point P117 (7.5, -320.5)
  point P118 (7.5, -320.5)
  point P119 (19.25, -320.5)
  point P120 (19.25, -320.5)
  point P121 (31, -320.5)
  point P122 (31, -320.5)
  point P123 (42.75, -320.5)
  point P124 (42.75, -320.5)
  point P125 (54.5, -320.5)
  point P126 (54.5, -320.5)
  point P127 (66.25, -320.5)
  point P128 (66.25, -320.5)
  point P129 (78, -320.5)
  point P130 (78, -320.5)
  point P131 (89.75, -320.5)
  point P132 (89.75, -320.5)
  point P133 (101.5, -320.5)
  point P134 (101.5, -320.5)
  point P135 (113.25, -320.5)
  point P136 (113.25, -320.5)
  point P137 (125, -320.5)
  point P138 (125, -320.5)
  point P139 (136.75, -320.5)
  point P140 (136.75, -320.5)
  point P141 (148.5, -320.5)
  point P142 (148.5, -320.5)
  point P143 (160.25, -320.5)
  point P144 (160.25, -320.5)
  point P145 (172, -320.5)
  point P146 (172, -320.5)
  point P147 (183.75, -320.5)
  point P148 (183.75, -320.5)
  point P149 (195.5, -320.5)
  point P150 (195.5, -320.5)
  point P151 (207.25, -320.5)
  point P152 (207.25, -320.5)
  point P153 (-67.5, -239.5)
  point P154 (242.5, -265.5)
  point P155 (242.5, -265.5)
  point P156 (219, -274.6667)
  point P157 (219, -274.6667)
  point P158 (242.5, -274.6667)
  point P159 (242.5, -274.6667)
  point P160 (219, -283.8333)
  point P161 (219, -283.8333)
  point P162 (242.5, -283.8333)
  point P163 (242.5, -283.8333)
  point P164 (219, -293)
  point P165 (219, -293)
  point P166 (230.75, -293)
  point P167 (230.75, -293)
  point P168 (242.5, -293)
  point P169 (242.5, -293)
  point P170 (219, -302.1667)
  point P171 (219, -302.1667)
  point P172 (230.75, -302.1667)
  point P173 (230.75, -302.1667)
  point P174 (242.5, -302.1667)
  point P175 (242.5, -302.1667)
  point P176 (219, -311.3333)
  point P177 (219, -311.3333)
  point P178 (230.75, -311.3333)